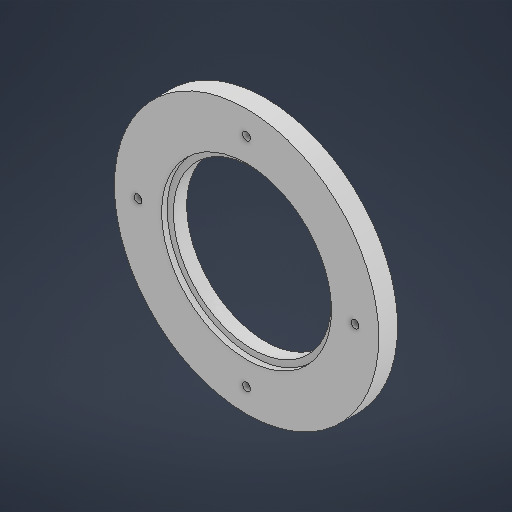
# Autodesk Inventor part: Fix_bearing_Base
Saved by Autodesk Inventor 2025.2 (Build 292293000, 293)
## iProperties
Created: 2025-07-10
Part Number: Fix_bearing_Base
Material: Generic
Document SubType Name: Modeling
Designer: Tiago
Density: 1 g/cm^3
Appearance: Default
Author: Tiago
Autodesk Inventor part; units mm, degrees
ref_plane "YZ Plane" through (0, 0, 0) normal (1, 0, 0) x (0, 1, 0)
ref_plane "XZ Plane" through (0, 0, 0) normal (0, 1, 0) x (-1, 0, 0)
ref_plane "XY Plane" through (0, 0, 0) normal (0, 0, 1) x (1, 0, 0)
sketch "Sketch1" plane through (0, 0, 0) normal (0, 0, 1) x (1, 0, 0)
  circle A0 centre (0, 0) radius 45
  circle A1 centre (0, 0) radius 57.417 construction
  circle A2 centre (-57.417, 0) radius 2.1
  circle A3 centre (0, -57.417) radius 2.1
  circle A4 centre (57.417, 0) radius 2.1
  circle A5 centre (0, 57.417) radius 2.1
  circle A6 centre (0, 0) radius 70
  circle A7 centre (0, 0) radius 41.75
  dimension "d1" = 114.834
  dimension "d0" = 90
  dimension "d2" = 4.2
  dimension "d5" = 360
  dimension "d7" = 140
  dimension "d8" = 83.5
  constraints: 7 centre point, 4 coincident, 2 horizontal alignment, 11 other
  measures "d0" diameter of A0
  measures "d2" diameter of A2
  measures "d7" diameter of A6
  measures "d8" diameter of A7
extrude "Extrusion1" add sketch "Sketch1" along normal blind 10 contours A6
extrude "Extrusion2" add sketch "Sketch1" along normal blind 7 contours A0
body "Solid1"
